Autodesk Inventor part; units mm, degrees
(part 2 of 3)
  line L952 (4.2416, 3.358) -> (4.3453, 3.3717)
  arc A20 (4.5494, 3.0907) -> (4.3453, 3.3717) centre (0, 0) ccw
  line L953 (4.5494, 3.0907) -> (4.5044, 2.9964)
  line L954 (4.5044, 2.9964) -> (4.4538, 2.9006)
  line L955 (4.4538, 2.9006) -> (4.403, 2.8135)
  line L956 (4.403, 2.8135) -> (4.3541, 2.7371)
  line L957 (4.3541, 2.7371) -> (4.3057, 2.6681)
  line L958 (4.3057, 2.6681) -> (4.2604, 2.609)
  line L959 (4.2604, 2.609) -> (4.2171, 2.5571)
  line L960 (4.2171, 2.5571) -> (4.1777, 2.5137)
  line L961 (4.1777, 2.5137) -> (4.1429, 2.4785)
  line L962 (4.1429, 2.4785) -> (4.0862, 2.4275)
  line L963 (4.0862, 2.4275) -> (4.0491, 2.3994)
  line L964 (4.0491, 2.3994) -> (3.9753, 2.3516)
  line L965 (3.9753, 2.3516) -> (3.9286, 2.314)
  line L966 (3.9286, 2.314) -> (3.9091, 2.2954)
  line L967 (3.9091, 2.2954) -> (3.892, 2.277)
  line L968 (3.892, 2.277) -> (3.8773, 2.2589)
  line L969 (3.8773, 2.2589) -> (3.8652, 2.2413)
  line L970 (3.8652, 2.2413) -> (3.8554, 2.2242)
  line L971 (3.8554, 2.2242) -> (3.8481, 2.2077)
  line L972 (3.8481, 2.2077) -> (3.8431, 2.1919)
  line L973 (3.8431, 2.1919) -> (3.8404, 2.1769)
  line L974 (3.8404, 2.1769) -> (3.8401, 2.1628)
  line L975 (3.8401, 2.1628) -> (3.842, 2.1497)
  line L976 (3.842, 2.1497) -> (3.8489, 2.1321)
  line L977 (3.8489, 2.1321) -> (3.9204, 1.9976)
  line L978 (3.9204, 1.9976) -> (3.9872, 1.8607)
  line L979 (3.9872, 1.8607) -> (3.9974, 1.8447)
  line L980 (3.9974, 1.8447) -> (4.0069, 1.8354)
  line L981 (4.0069, 1.8354) -> (4.0185, 1.8274)
  line L982 (4.0185, 1.8274) -> (4.0322, 1.8208)
  line L983 (4.0322, 1.8208) -> (4.0479, 1.8155)
  line L984 (4.0479, 1.8155) -> (4.0655, 1.8118)
  line L985 (4.0655, 1.8118) -> (4.0851, 1.8096)
  line L986 (4.0851, 1.8096) -> (4.1065, 1.8091)
  line L987 (4.1065, 1.8091) -> (4.1297, 1.8103)
  line L988 (4.1297, 1.8103) -> (4.1547, 1.8133)
  line L989 (4.1547, 1.8133) -> (4.1813, 1.8182)
  line L990 (4.1813, 1.8182) -> (4.2391, 1.8339)
  line L991 (4.2391, 1.8339) -> (4.3212, 1.8655)
  line L992 (4.3212, 1.8655) -> (4.3657, 1.879)
  line L993 (4.3657, 1.879) -> (4.4403, 1.8949)
  line L994 (4.4403, 1.8949) -> (4.4892, 1.9023)
  line L995 (4.4892, 1.9023) -> (4.5475, 1.9087)
  line L996 (4.5475, 1.9087) -> (4.6149, 1.9132)
  line L997 (4.6149, 1.9132) -> (4.6893, 1.9151)
  line L998 (4.6893, 1.9151) -> (4.7736, 1.9137)
  line L999 (4.7736, 1.9137) -> (4.8642, 1.9084)
  line L1000 (4.8642, 1.9084) -> (4.9645, 1.8983)
  line L1001 (4.9645, 1.8983) -> (5.0717, 1.8829)
  line L1002 (5.0717, 1.8829) -> (5.1745, 1.8639)
  arc A21 (5.2818, 1.5336) -> (5.1745, 1.8639) centre (0, 0) ccw
  line L1003 (5.2818, 1.5336) -> (5.2098, 1.4578)
  line L1004 (5.2098, 1.4578) -> (5.1322, 1.3823)
  line L1005 (5.1322, 1.3823) -> (5.0569, 1.3152)
  line L1006 (5.0569, 1.3152) -> (4.9868, 1.2577)
  line L1007 (4.9868, 1.2577) -> (4.9194, 1.207)
  line L1008 (4.9194, 1.207) -> (4.8581, 1.1647)
  line L1009 (4.8581, 1.1647) -> (4.8009, 1.1288)
  line L1010 (4.8009, 1.1288) -> (4.75, 1.0997)
  line L1011 (4.75, 1.0997) -> (4.7061, 1.0769)
  line L1012 (4.7061, 1.0769) -> (4.6364, 1.046)
  line L1013 (4.6364, 1.046) -> (4.5924, 1.0307)
  line L1014 (4.5924, 1.0307) -> (4.5075, 1.0081)
  line L1015 (4.5075, 1.0081) -> (4.4514, 0.9867)
  line L1016 (4.4514, 0.9867) -> (4.427, 0.9751)
  line L1017 (4.427, 0.9751) -> (4.4051, 0.9628)
  line L1018 (4.4051, 0.9628) -> (4.3856, 0.9502)
  line L1019 (4.3856, 0.9502) -> (4.3686, 0.9372)
  line L1020 (4.3686, 0.9372) -> (4.354, 0.9239)
  line L1021 (4.354, 0.9239) -> (4.3419, 0.9105)
  line L1022 (4.3419, 0.9105) -> (4.3323, 0.897)
  line L1023 (4.3323, 0.897) -> (4.3252, 0.8836)
  line L1024 (4.3252, 0.8836) -> (4.3205, 0.8703)
  line L1025 (4.3205, 0.8703) -> (4.3182, 0.8572)
  line L1026 (4.3182, 0.8572) -> (4.3194, 0.8383)
  line L1027 (4.3194, 0.8383) -> (4.3458, 0.6883)
  line L1028 (4.3458, 0.6883) -> (4.3671, 0.5375)
  line L1029 (4.3671, 0.5375) -> (4.3718, 0.5191)
  line L1030 (4.3718, 0.5191) -> (4.378, 0.5074)
  line L1031 (4.378, 0.5074) -> (4.3865, 0.4962)
  line L1032 (4.3865, 0.4962) -> (4.3975, 0.4856)
  line L1033 (4.3975, 0.4856) -> (4.4108, 0.4758)
  line L1034 (4.4108, 0.4758) -> (4.4264, 0.4668)
  line L1035 (4.4264, 0.4668) -> (4.4444, 0.4587)
  line L1036 (4.4444, 0.4587) -> (4.4646, 0.4516)
  line L1037 (4.4646, 0.4516) -> (4.487, 0.4455)
  line L1038 (4.487, 0.4455) -> (4.5117, 0.4407)
  line L1039 (4.5117, 0.4407) -> (4.5385, 0.4371)
  line L1040 (4.5385, 0.4371) -> (4.5984, 0.4341)
  line L1041 (4.5984, 0.4341) -> (4.6862, 0.4388)
  line L1042 (4.6862, 0.4388) -> (4.7327, 0.438)
  line L1043 (4.7327, 0.438) -> (4.8085, 0.43)
  line L1044 (4.8085, 0.43) -> (4.8574, 0.422)
  line L1045 (4.8574, 0.422) -> (4.9147, 0.41)
  line L1046 (4.9147, 0.41) -> (4.9802, 0.3935)
  line L1047 (4.9802, 0.3935) -> (5.0516, 0.3723)
  line L1048 (5.0516, 0.3723) -> (5.1313, 0.3449)
  line L1049 (5.1313, 0.3449) -> (5.2159, 0.3118)
  line L1050 (5.2159, 0.3118) -> (5.3081, 0.2712)
  line L1051 (5.3081, 0.2712) -> (5.4053, 0.2235)
  line L1052 (5.4053, 0.2235) -> (5.4973, 0.1736)
  arc A22 (5.4973, -0.1736) -> (5.4973, 0.1736) centre (0, 0) ccw
  line L1053 (5.4973, -0.1736) -> (5.4053, -0.2235)
  line L1054 (5.4053, -0.2235) -> (5.3081, -0.2712)
  line L1055 (5.3081, -0.2712) -> (5.2159, -0.3118)
  line L1056 (5.2159, -0.3118) -> (5.1313, -0.3449)
  line L1057 (5.1313, -0.3449) -> (5.0516, -0.3723)
  line L1058 (5.0516, -0.3723) -> (4.9802, -0.3935)
  line L1059 (4.9802, -0.3935) -> (4.9147, -0.41)
  line L1060 (4.9147, -0.41) -> (4.8574, -0.422)
  line L1061 (4.8574, -0.422) -> (4.8085, -0.43)
  line L1062 (4.8085, -0.43) -> (4.7327, -0.438)
  line L1063 (4.7327, -0.438) -> (4.6862, -0.4388)
  line L1064 (4.6862, -0.4388) -> (4.5984, -0.4341)
  line L1065 (4.5984, -0.4341) -> (4.5385, -0.4371)
  line L1066 (4.5385, -0.4371) -> (4.5117, -0.4407)
  line L1067 (4.5117, -0.4407) -> (4.487, -0.4455)
  line L1068 (4.487, -0.4455) -> (4.4646, -0.4516)
  line L1069 (4.4646, -0.4516) -> (4.4444, -0.4587)
  line L1070 (4.4444, -0.4587) -> (4.4264, -0.4668)
  line L1071 (4.4264, -0.4668) -> (4.4108, -0.4758)
  line L1072 (4.4108, -0.4758) -> (4.3975, -0.4856)
  line L1073 (4.3975, -0.4856) -> (4.3865, -0.4962)
  line L1074 (4.3865, -0.4962) -> (4.378, -0.5074)
  line L1075 (4.378, -0.5074) -> (4.3718, -0.5191)
  line L1076 (4.3718, -0.5191) -> (4.3671, -0.5375)
  line L1077 (4.3671, -0.5375) -> (4.3458, -0.6883)
  line L1078 (4.3458, -0.6883) -> (4.3194, -0.8383)
  line L1079 (4.3194, -0.8383) -> (4.3182, -0.8572)
  line L1080 (4.3182, -0.8572) -> (4.3205, -0.8703)
  line L1081 (4.3205, -0.8703) -> (4.3252, -0.8836)
  line L1082 (4.3252, -0.8836) -> (4.3323, -0.897)
  line L1083 (4.3323, -0.897) -> (4.3419, -0.9105)
  line L1084 (4.3419, -0.9105) -> (4.354, -0.9239)
  line L1085 (4.354, -0.9239) -> (4.3686, -0.9372)
  line L1086 (4.3686, -0.9372) -> (4.3856, -0.9502)
  line L1087 (4.3856, -0.9502) -> (4.4051, -0.9628)
  line L1088 (4.4051, -0.9628) -> (4.427, -0.9751)
  line L1089 (4.427, -0.9751) -> (4.4514, -0.9867)
  line L1090 (4.4514, -0.9867) -> (4.5075, -1.0081)
  line L1091 (4.5075, -1.0081) -> (4.5924, -1.0307)
  line L1092 (4.5924, -1.0307) -> (4.6364, -1.046)
  line L1093 (4.6364, -1.046) -> (4.7061, -1.0769)
  line L1094 (4.7061, -1.0769) -> (4.75, -1.0997)
  line L1095 (4.75, -1.0997) -> (4.8009, -1.1288)
  line L1096 (4.8009, -1.1288) -> (4.8581, -1.1647)
  line L1097 (4.8581, -1.1647) -> (4.9194, -1.207)
  line L1098 (4.9194, -1.207) -> (4.9868, -1.2577)
  line L1099 (4.9868, -1.2577) -> (5.0569, -1.3152)
  line L1100 (5.0569, -1.3152) -> (5.1322, -1.3823)
  line L1101 (5.1322, -1.3823) -> (5.2098, -1.4578)
  line L1102 (5.2098, -1.4578) -> (5.2818, -1.5336)
  arc A23 (5.1745, -1.8639) -> (5.2818, -1.5336) centre (0, 0) ccw
  line L1103 (5.1745, -1.8639) -> (5.0717, -1.8829)
  line L1104 (5.0717, -1.8829) -> (4.9645, -1.8983)
  line L1105 (4.9645, -1.8983) -> (4.8642, -1.9084)
  line L1106 (4.8642, -1.9084) -> (4.7736, -1.9137)
  line L1107 (4.7736, -1.9137) -> (4.6893, -1.9151)
  line L1108 (4.6893, -1.9151) -> (4.6149, -1.9132)
  line L1109 (4.6149, -1.9132) -> (4.5475, -1.9087)
  line L1110 (4.5475, -1.9087) -> (4.4892, -1.9023)
  line L1111 (4.4892, -1.9023) -> (4.4403, -1.8949)
  line L1112 (4.4403, -1.8949) -> (4.3657, -1.879)
  line L1113 (4.3657, -1.879) -> (4.3212, -1.8655)
  line L1114 (4.3212, -1.8655) -> (4.2391, -1.8339)
  line L1115 (4.2391, -1.8339) -> (4.1813, -1.8182)
  line L1116 (4.1813, -1.8182) -> (4.1547, -1.8133)
  line L1117 (4.1547, -1.8133) -> (4.1297, -1.8103)
  line L1118 (4.1297, -1.8103) -> (4.1065, -1.8091)
  line L1119 (4.1065, -1.8091) -> (4.0851, -1.8096)
  line L1120 (4.0851, -1.8096) -> (4.0655, -1.8118)
  line L1121 (4.0655, -1.8118) -> (4.0479, -1.8155)
  line L1122 (4.0479, -1.8155) -> (4.0322, -1.8208)
  line L1123 (4.0322, -1.8208) -> (4.0185, -1.8274)
  line L1124 (4.0185, -1.8274) -> (4.0069, -1.8354)
  line L1125 (4.0069, -1.8354) -> (3.9974, -1.8447)
  line L1126 (3.9974, -1.8447) -> (3.9872, -1.8607)
  line L1127 (3.9872, -1.8607) -> (3.9204, -1.9976)
  line L1128 (3.9204, -1.9976) -> (3.8489, -2.1321)
  line L1129 (3.8489, -2.1321) -> (3.842, -2.1497)
  line L1130 (3.842, -2.1497) -> (3.8401, -2.1628)
  line L1131 (3.8401, -2.1628) -> (3.8404, -2.1769)
  line L1132 (3.8404, -2.1769) -> (3.8431, -2.1919)
  line L1133 (3.8431, -2.1919) -> (3.8481, -2.2077)
  line L1134 (3.8481, -2.2077) -> (3.8554, -2.2242)
  line L1135 (3.8554, -2.2242) -> (3.8652, -2.2413)
  line L1136 (3.8652, -2.2413) -> (3.8773, -2.2589)
  line L1137 (3.8773, -2.2589) -> (3.892, -2.277)
  line L1138 (3.892, -2.277) -> (3.9091, -2.2954)
  line L1139 (3.9091, -2.2954) -> (3.9286, -2.314)
  line L1140 (3.9286, -2.314) -> (3.9753, -2.3516)
  line L1141 (3.9753, -2.3516) -> (4.0491, -2.3994)
  line L1142 (4.0491, -2.3994) -> (4.0862, -2.4275)
  line L1143 (4.0862, -2.4275) -> (4.1429, -2.4785)
  line L1144 (4.1429, -2.4785) -> (4.1777, -2.5137)
  line L1145 (4.1777, -2.5137) -> (4.2171, -2.5571)
  line L1146 (4.2171, -2.5571) -> (4.2604, -2.609)
  line L1147 (4.2604, -2.609) -> (4.3057, -2.6681)
  line L1148 (4.3057, -2.6681) -> (4.3541, -2.7371)
  line L1149 (4.3541, -2.7371) -> (4.403, -2.8135)
  line L1150 (4.403, -2.8135) -> (4.4538, -2.9006)
  line L1151 (4.4538, -2.9006) -> (4.5044, -2.9964)
  line L1152 (4.5044, -2.9964) -> (4.5494, -3.0907)
  arc A24 (4.3453, -3.3717) -> (4.5494, -3.0907) centre (0, 0) ccw
  line L1153 (4.3453, -3.3717) -> (4.2416, -3.358)
  line L1154 (4.2416, -3.358) -> (4.1349, -3.3395)
  line L1155 (4.1349, -3.3395) -> (4.0364, -3.3181)
  line L1156 (4.0364, -3.3181) -> (3.9486, -3.2952)
  line L1157 (3.9486, -3.2952) -> (3.868, -3.2704)
  line L1158 (3.868, -3.2704) -> (3.7978, -3.2457)
  line L1159 (3.7978, -3.2457) -> (3.7351, -3.2205)
  line L1160 (3.7351, -3.2205) -> (3.6817, -3.1965)
  line L1161 (3.6817, -3.1965) -> (3.6374, -3.1743)
  line L1162 (3.6374, -3.1743) -> (3.5714, -3.1361)
  line L1163 (3.5714, -3.1361) -> (3.5332, -3.1095)
  line L1164 (3.5332, -3.1095) -> (3.465, -3.0541)
  line L1165 (3.465, -3.0541) -> (3.4148, -3.0213)
  line L1166 (3.4148, -3.0213) -> (3.391, -3.0084)
  line L1167 (3.391, -3.0084) -> (3.3682, -2.9979)
  line L1168 (3.3682, -2.9979) -> (3.3465, -2.9895)
  line L1169 (3.3465, -2.9895) -> (3.326, -2.9834)
  line L1170 (3.326, -2.9834) -> (3.3067, -2.9794)
  line L1171 (3.3067, -2.9794) -> (3.2887, -2.9775)
  line L1172 (3.2887, -2.9775) -> (3.2722, -2.9777)
  line L1173 (3.2722, -2.9777) -> (3.2571, -2.9798)
  line L1174 (3.2571, -2.9798) -> (3.2436, -2.9838)
  line L1175 (3.2436, -2.9838) -> (3.2317, -2.9896)
  line L1176 (3.2317, -2.9896) -> (3.2171, -3.0017)
  line L1177 (3.2171, -3.0017) -> (3.1113, -3.1113)
  line L1178 (3.1113, -3.1113) -> (3.0017, -3.2171)
  line L1179 (3.0017, -3.2171) -> (2.9896, -3.2317)
  line L1180 (2.9896, -3.2317) -> (2.9838, -3.2436)
  line L1181 (2.9838, -3.2436) -> (2.9798, -3.2571)
  line L1182 (2.9798, -3.2571) -> (2.9777, -3.2722)
  line L1183 (2.9777, -3.2722) -> (2.9775, -3.2887)
  line L1184 (2.9775, -3.2887) -> (2.9794, -3.3067)
  line L1185 (2.9794, -3.3067) -> (2.9834, -3.326)
  line L1186 (2.9834, -3.326) -> (2.9895, -3.3465)
  line L1187 (2.9895, -3.3465) -> (2.9979, -3.3682)
  line L1188 (2.9979, -3.3682) -> (3.0084, -3.391)
  line L1189 (3.0084, -3.391) -> (3.0213, -3.4148)
  line L1190 (3.0213, -3.4148) -> (3.0541, -3.465)
  line L1191 (3.0541, -3.465) -> (3.1095, -3.5332)
  line L1192 (3.1095, -3.5332) -> (3.1361, -3.5714)
  line L1193 (3.1361, -3.5714) -> (3.1743, -3.6374)
  line L1194 (3.1743, -3.6374) -> (3.1965, -3.6817)
  line L1195 (3.1965, -3.6817) -> (3.2205, -3.7351)
  line L1196 (3.2205, -3.7351) -> (3.2457, -3.7978)
  line L1197 (3.2457, -3.7978) -> (3.2704, -3.868)
  line L1198 (3.2704, -3.868) -> (3.2952, -3.9486)
  line L1199 (3.2952, -3.9486) -> (3.3181, -4.0364)
  line L1200 (3.3181, -4.0364) -> (3.3395, -4.1349)
  line L1201 (3.3395, -4.1349) -> (3.358, -4.2416)
  line L1202 (3.358, -4.2416) -> (3.3717, -4.3453)
  arc A25 (3.0907, -4.5494) -> (3.3717, -4.3453) centre (0, 0) ccw
  line L1203 (3.0907, -4.5494) -> (2.9964, -4.5044)
  line L1204 (2.9964, -4.5044) -> (2.9006, -4.4538)
  line L1205 (2.9006, -4.4538) -> (2.8135, -4.403)
  line L1206 (2.8135, -4.403) -> (2.7371, -4.3541)
  line L1207 (2.7371, -4.3541) -> (2.6681, -4.3057)
  line L1208 (2.6681, -4.3057) -> (2.609, -4.2604)
  line L1209 (2.609, -4.2604) -> (2.5571, -4.2171)
  line L1210 (2.5571, -4.2171) -> (2.5137, -4.1777)
  line L1211 (2.5137, -4.1777) -> (2.4785, -4.1429)
  line L1212 (2.4785, -4.1429) -> (2.4275, -4.0862)
  line L1213 (2.4275, -4.0862) -> (2.3994, -4.0491)
  line L1214 (2.3994, -4.0491) -> (2.3516, -3.9753)
  line L1215 (2.3516, -3.9753) -> (2.314, -3.9286)
  line L1216 (2.314, -3.9286) -> (2.2954, -3.9091)
  line L1217 (2.2954, -3.9091) -> (2.277, -3.892)
  line L1218 (2.277, -3.892) -> (2.2589, -3.8773)
  line L1219 (2.2589, -3.8773) -> (2.2413, -3.8652)
  line L1220 (2.2413, -3.8652) -> (2.2242, -3.8554)
  line L1221 (2.2242, -3.8554) -> (2.2077, -3.8481)
  line L1222 (2.2077, -3.8481) -> (2.1919, -3.8431)
  line L1223 (2.1919, -3.8431) -> (2.1769, -3.8404)
  line L1224 (2.1769, -3.8404) -> (2.1628, -3.8401)
  line L1225 (2.1628, -3.8401) -> (2.1497, -3.842)
  line L1226 (2.1497, -3.842) -> (2.1321, -3.8489)
  line L1227 (2.1321, -3.8489) -> (1.9976, -3.9204)
  line L1228 (1.9976, -3.9204) -> (1.8607, -3.9872)
  line L1229 (1.8607, -3.9872) -> (1.8447, -3.9974)
  line L1230 (1.8447, -3.9974) -> (1.8354, -4.0069)
  line L1231 (1.8354, -4.0069) -> (1.8274, -4.0185)
  line L1232 (1.8274, -4.0185) -> (1.8208, -4.0322)
  line L1233 (1.8208, -4.0322) -> (1.8155, -4.0479)
  line L1234 (1.8155, -4.0479) -> (1.8118, -4.0655)
  line L1235 (1.8118, -4.0655) -> (1.8096, -4.0851)
  line L1236 (1.8096, -4.0851) -> (1.8091, -4.1065)
  line L1237 (1.8091, -4.1065) -> (1.8103, -4.1297)
  line L1238 (1.8103, -4.1297) -> (1.8133, -4.1547)
  line L1239 (1.8133, -4.1547) -> (1.8182, -4.1813)
  line L1240 (1.8182, -4.1813) -> (1.8339, -4.2391)
  line L1241 (1.8339, -4.2391) -> (1.8655, -4.3212)
  line L1242 (1.8655, -4.3212) -> (1.879, -4.3657)
  line L1243 (1.879, -4.3657) -> (1.8949, -4.4403)
  line L1244 (1.8949, -4.4403) -> (1.9023, -4.4892)
  line L1245 (1.9023, -4.4892) -> (1.9087, -4.5475)
  line L1246 (1.9087, -4.5475) -> (1.9132, -4.6149)
  line L1247 (1.9132, -4.6149) -> (1.9151, -4.6893)
  line L1248 (1.9151, -4.6893) -> (1.9137, -4.7736)
  line L1249 (1.9137, -4.7736) -> (1.9084, -4.8642)
  line L1250 (1.9084, -4.8642) -> (1.8983, -4.9645)
  line L1251 (1.8983, -4.9645) -> (1.8829, -5.0717)
  line L1252 (1.8829, -5.0717) -> (1.8639, -5.1745)
  arc A26 (1.5336, -5.2818) -> (1.8639, -5.1745) centre (0, 0) ccw
  line L1253 (1.5336, -5.2818) -> (1.4578, -5.2098)
  line L1254 (1.4578, -5.2098) -> (1.3823, -5.1322)
  line L1255 (1.3823, -5.1322) -> (1.3152, -5.0569)
  line L1256 (1.3152, -5.0569) -> (1.2577, -4.9868)
  line L1257 (1.2577, -4.9868) -> (1.207, -4.9194)
  line L1258 (1.207, -4.9194) -> (1.1647, -4.8581)
  line L1259 (1.1647, -4.8581) -> (1.1288, -4.8009)
  line L1260 (1.1288, -4.8009) -> (1.0997, -4.75)
  line L1261 (1.0997, -4.75) -> (1.0769, -4.7061)
  line L1262 (1.0769, -4.7061) -> (1.046, -4.6364)
  line L1263 (1.046, -4.6364) -> (1.0307, -4.5924)
  line L1264 (1.0307, -4.5924) -> (1.0081, -4.5075)
  line L1265 (1.0081, -4.5075) -> (0.9867, -4.4514)
  line L1266 (0.9867, -4.4514) -> (0.9751, -4.427)
  line L1267 (0.9751, -4.427) -> (0.9628, -4.4051)
  line L1268 (0.9628, -4.4051) -> (0.9502, -4.3856)
  line L1269 (0.9502, -4.3856) -> (0.9372, -4.3686)
  line L1270 (0.9372, -4.3686) -> (0.9239, -4.354)
  line L1271 (0.9239, -4.354) -> (0.9105, -4.3419)
  line L1272 (0.9105, -4.3419) -> (0.897, -4.3323)
  line L1273 (0.897, -4.3323) -> (0.8836, -4.3252)
  line L1274 (0.8836, -4.3252) -> (0.8703, -4.3205)
  line L1275 (0.8703, -4.3205) -> (0.8572, -4.3182)
  line L1276 (0.8572, -4.3182) -> (0.8383, -4.3194)
  line L1277 (0.8383, -4.3194) -> (0.6883, -4.3458)
  line L1278 (0.6883, -4.3458) -> (0.5375, -4.3671)
  line L1279 (0.5375, -4.3671) -> (0.5191, -4.3718)
  line L1280 (0.5191, -4.3718) -> (0.5074, -4.378)
  line L1281 (0.5074, -4.378) -> (0.4962, -4.3865)
  line L1282 (0.4962, -4.3865) -> (0.4856, -4.3975)
  line L1283 (0.4856, -4.3975) -> (0.4758, -4.4108)
  line L1284 (0.4758, -4.4108) -> (0.4668, -4.4264)
  line L1285 (0.4668, -4.4264) -> (0.4587, -4.4444)
  line L1286 (0.4587, -4.4444) -> (0.4516, -4.4646)
  line L1287 (0.4516, -4.4646) -> (0.4455, -4.487)
  line L1288 (0.4455, -4.487) -> (0.4407, -4.5117)
  line L1289 (0.4407, -4.5117) -> (0.4371, -4.5385)
  line L1290 (0.4371, -4.5385) -> (0.4341, -4.5984)
  line L1291 (0.4341, -4.5984) -> (0.4388, -4.6862)
  line L1292 (0.4388, -4.6862) -> (0.438, -4.7327)
  line L1293 (0.438, -4.7327) -> (0.43, -4.8085)
  line L1294 (0.43, -4.8085) -> (0.422, -4.8574)
  line L1295 (0.422, -4.8574) -> (0.41, -4.9147)
  line L1296 (0.41, -4.9147) -> (0.3935, -4.9802)
  line L1297 (0.3935, -4.9802) -> (0.3723, -5.0516)
  line L1298 (0.3723, -5.0516) -> (0.3449, -5.1313)
  line L1299 (0.3449, -5.1313) -> (0.3118, -5.2159)
  line L1300 (0.3118, -5.2159) -> (0.2712, -5.3081)
  line L1301 (0.2712, -5.3081) -> (0.2235, -5.4053)
  line L1302 (0.2235, -5.4053) -> (0.1736, -5.4973)
  arc A27 (-0.1736, -5.4973) -> (0.1736, -5.4973) centre (0, 0) ccw
  line L1303 (-0.1736, -5.4973) -> (-0.2235, -5.4053)
  line L1304 (-0.2235, -5.4053) -> (-0.2712, -5.3081)
  line L1305 (-0.2712, -5.3081) -> (-0.3118, -5.2159)
  line L1306 (-0.3118, -5.2159) -> (-0.3449, -5.1313)
  line L1307 (-0.3449, -5.1313) -> (-0.3723, -5.0516)
  line L1308 (-0.3723, -5.0516) -> (-0.3935, -4.9802)
  line L1309 (-0.3935, -4.9802) -> (-0.41, -4.9147)
  line L1310 (-0.41, -4.9147) -> (-0.422, -4.8574)
  line L1311 (-0.422, -4.8574) -> (-0.43, -4.8085)
  line L1312 (-0.43, -4.8085) -> (-0.438, -4.7327)
  line L1313 (-0.438, -4.7327) -> (-0.4388, -4.6862)
  line L1314 (-0.4388, -4.6862) -> (-0.4341, -4.5984)
  line L1315 (-0.4341, -4.5984) -> (-0.4371, -4.5385)
  line L1316 (-0.4371, -4.5385) -> (-0.4407, -4.5117)
  line L1317 (-0.4407, -4.5117) -> (-0.4455, -4.487)
  line L1318 (-0.4455, -4.487) -> (-0.4516, -4.4646)
  line L1319 (-0.4516, -4.4646) -> (-0.4587, -4.4444)
  line L1320 (-0.4587, -4.4444) -> (-0.4668, -4.4264)
  line L1321 (-0.4668, -4.4264) -> (-0.4758, -4.4108)
  line L1322 (-0.4758, -4.4108) -> (-0.4856, -4.3975)
  line L1323 (-0.4856, -4.3975) -> (-0.4962, -4.3865)
  line L1324 (-0.4962, -4.3865) -> (-0.5074, -4.378)
  line L1325 (-0.5074, -4.378) -> (-0.5191, -4.3718)
  line L1326 (-0.5191, -4.3718) -> (-0.5375, -4.3671)
  line L1327 (-0.5375, -4.3671) -> (-0.6883, -4.3458)
  line L1328 (-0.6883, -4.3458) -> (-0.8383, -4.3194)
  line L1329 (-0.8383, -4.3194) -> (-0.8572, -4.3182)
  line L1330 (-0.8572, -4.3182) -> (-0.8703, -4.3205)
  line L1331 (-0.8703, -4.3205) -> (-0.8836, -4.3252)
  line L1332 (-0.8836, -4.3252) -> (-0.897, -4.3323)
  line L1333 (-0.897, -4.3323) -> (-0.9105, -4.3419)
  line L1334 (-0.9105, -4.3419) -> (-0.9239, -4.354)
  line L1335 (-0.9239, -4.354) -> (-0.9372, -4.3686)
  line L1336 (-0.9372, -4.3686) -> (-0.9502, -4.3856)
  line L1337 (-0.9502, -4.3856) -> (-0.9628, -4.4051)
  line L1338 (-0.9628, -4.4051) -> (-0.9751, -4.427)
  line L1339 (-0.9751, -4.427) -> (-0.9867, -4.4514)
  line L1340 (-0.9867, -4.4514) -> (-1.0081, -4.5075)
  line L1341 (-1.0081, -4.5075) -> (-1.0307, -4.5924)
  line L1342 (-1.0307, -4.5924) -> (-1.046, -4.6364)
  line L1343 (-1.046, -4.6364) -> (-1.0769, -4.7061)
  line L1344 (-1.0769, -4.7061) -> (-1.0997, -4.75)
  line L1345 (-1.0997, -4.75) -> (-1.1288, -4.8009)
  line L1346 (-1.1288, -4.8009) -> (-1.1647, -4.8581)
  line L1347 (-1.1647, -4.8581) -> (-1.207, -4.9194)
  line L1348 (-1.207, -4.9194) -> (-1.2577, -4.9868)
  line L1349 (-1.2577, -4.9868) -> (-1.3152, -5.0569)
  line L1350 (-1.3152, -5.0569) -> (-1.3823, -5.1322)
  line L1351 (-1.3823, -5.1322) -> (-1.4578, -5.2098)
  line L1352 (-1.4578, -5.2098) -> (-1.5336, -5.2818)
  arc A28 (-1.8639, -5.1745) -> (-1.5336, -5.2818) centre (0, 0) ccw
  line L1353 (-1.8639, -5.1745) -> (-1.8829, -5.0717)
  line L1354 (-1.8829, -5.0717) -> (-1.8983, -4.9645)
  line L1355 (-1.8983, -4.9645) -> (-1.9084, -4.8642)
  line L1356 (-1.9084, -4.8642) -> (-1.9137, -4.7736)
  line L1357 (-1.9137, -4.7736) -> (-1.9151, -4.6893)
  line L1358 (-1.9151, -4.6893) -> (-1.9132, -4.6149)
  line L1359 (-1.9132, -4.6149) -> (-1.9087, -4.5475)
  line L1360 (-1.9087, -4.5475) -> (-1.9023, -4.4892)
  line L1361 (-1.9023, -4.4892) -> (-1.8949, -4.4403)
  line L1362 (-1.8949, -4.4403) -> (-1.879, -4.3657)
  line L1363 (-1.879, -4.3657) -> (-1.8655, -4.3212)
  line L1364 (-1.8655, -4.3212) -> (-1.8339, -4.2391)
  line L1365 (-1.8339, -4.2391) -> (-1.8182, -4.1813)
  line L1366 (-1.8182, -4.1813) -> (-1.8133, -4.1547)
  line L1367 (-1.8133, -4.1547) -> (-1.8103, -4.1297)
  line L1368 (-1.8103, -4.1297) -> (-1.8091, -4.1065)
  line L1369 (-1.8091, -4.1065) -> (-1.8096, -4.0851)
  line L1370 (-1.8096, -4.0851) -> (-1.8118, -4.0655)
  line L1371 (-1.8118, -4.0655) -> (-1.8155, -4.0479)
  line L1372 (-1.8155, -4.0479) -> (-1.8208, -4.0322)
  line L1373 (-1.8208, -4.0322) -> (-1.8274, -4.0185)
  line L1374 (-1.8274, -4.0185) -> (-1.8354, -4.0069)
  line L1375 (-1.8354, -4.0069) -> (-1.8447, -3.9974)
  line L1376 (-1.8447, -3.9974) -> (-1.8607, -3.9872)
  line L1377 (-1.8607, -3.9872) -> (-1.9976, -3.9204)
  line L1378 (-1.9976, -3.9204) -> (-2.1321, -3.8489)
  line L1379 (-2.1321, -3.8489) -> (-2.1497, -3.842)
  line L1380 (-2.1497, -3.842) -> (-2.1628, -3.8401)
  line L1381 (-2.1628, -3.8401) -> (-2.1769, -3.8404)
  line L1382 (-2.1769, -3.8404) -> (-2.1919, -3.8431)
  line L1383 (-2.1919, -3.8431) -> (-2.2077, -3.8481)
  line L1384 (-2.2077, -3.8481) -> (-2.2242, -3.8554)
  line L1385 (-2.2242, -3.8554) -> (-2.2413, -3.8652)
  line L1386 (-2.2413, -3.8652) -> (-2.2589, -3.8773)
  line L1387 (-2.2589, -3.8773) -> (-2.277, -3.892)
  line L1388 (-2.277, -3.892) -> (-2.2954, -3.9091)
  line L1389 (-2.2954, -3.9091) -> (-2.314, -3.9286)
  line L1390 (-2.314, -3.9286) -> (-2.3516, -3.9753)
  line L1391 (-2.3516, -3.9753) -> (-2.3994, -4.0491)
  line L1392 (-2.3994, -4.0491) -> (-2.4275, -4.0862)
  line L1393 (-2.4275, -4.0862) -> (-2.4785, -4.1429)
  line L1394 (-2.4785, -4.1429) -> (-2.5137, -4.1777)
  line L1395 (-2.5137, -4.1777) -> (-2.5571, -4.2171)
  line L1396 (-2.5571, -4.2171) -> (-2.609, -4.2604)
  line L1397 (-2.609, -4.2604) -> (-2.6681, -4.3057)
  line L1398 (-2.6681, -4.3057) -> (-2.7371, -4.3541)
  line L1399 (-2.7371, -4.3541) -> (-2.8135, -4.403)
  line L1400 (-2.8135, -4.403) -> (-2.9006, -4.4538)
  line L1401 (-2.9006, -4.4538) -> (-2.9964, -4.5044)
  line L1402 (-2.9964, -4.5044) -> (-3.0907, -4.5494)
  arc A29 (-3.3717, -4.3453) -> (-3.0907, -4.5494) centre (0, 0) ccw
  line L1403 (-3.3717, -4.3453) -> (-3.358, -4.2416)
  line L1404 (-3.358, -4.2416) -> (-3.3395, -4.1349)
  line L1405 (-3.3395, -4.1349) -> (-3.3181, -4.0364)
  line L1406 (-3.3181, -4.0364) -> (-3.2952, -3.9486)
  line L1407 (-3.2952, -3.9486) -> (-3.2704, -3.868)
  line L1408 (-3.2704, -3.868) -> (-3.2457, -3.7978)
  line L1409 (-3.2457, -3.7978) -> (-3.2205, -3.7351)
  line L1410 (-3.2205, -3.7351) -> (-3.1965, -3.6817)
  line L1411 (-3.1965, -3.6817) -> (-3.1743, -3.6374)
  line L1412 (-3.1743, -3.6374) -> (-3.1361, -3.5714)
  line L1413 (-3.1361, -3.5714) -> (-3.1095, -3.5332)
  line L1414 (-3.1095, -3.5332) -> (-3.0541, -3.465)
  line L1415 (-3.0541, -3.465) -> (-3.0213, -3.4148)
  line L1416 (-3.0213, -3.4148) -> (-3.0084, -3.391)
  line L1417 (-3.0084, -3.391) -> (-2.9979, -3.3682)
  line L1418 (-2.9979, -3.3682) -> (-2.9895, -3.3465)
  line L1419 (-2.9895, -3.3465) -> (-2.9834, -3.326)
  line L1420 (-2.9834, -3.326) -> (-2.9794, -3.3067)
  line L1421 (-2.9794, -3.3067) -> (-2.9775, -3.2887)
  line L1422 (-2.9775, -3.2887) -> (-2.9777, -3.2722)
  line L1423 (-2.9777, -3.2722) -> (-2.9798, -3.2571)
  line L1424 (-2.9798, -3.2571) -> (-2.9838, -3.2436)
  line L1425 (-2.9838, -3.2436) -> (-2.9896, -3.2317)
  line L1426 (-2.9896, -3.2317) -> (-3.0017, -3.2171)
  line L1427 (-3.0017, -3.2171) -> (-3.1113, -3.1113)
  line L1428 (-3.1113, -3.1113) -> (-3.2171, -3.0017)
  line L1429 (-3.2171, -3.0017) -> (-3.2317, -2.9896)
  line L1430 (-3.2317, -2.9896) -> (-3.2436, -2.9838)
  line L1431 (-3.2436, -2.9838) -> (-3.2571, -2.9798)
  line L1432 (-3.2571, -2.9798) -> (-3.2722, -2.9777)
  line L1433 (-3.2722, -2.9777) -> (-3.2887, -2.9775)
  line L1434 (-3.2887, -2.9775) -> (-3.3067, -2.9794)
  line L1435 (-3.3067, -2.9794) -> (-3.326, -2.9834)
  line L1436 (-3.326, -2.9834) -> (-3.3465, -2.9895)
  line L1437 (-3.3465, -2.9895) -> (-3.3682, -2.9979)
  line L1438 (-3.3682, -2.9979) -> (-3.391, -3.0084)
  line L1439 (-3.391, -3.0084) -> (-3.4148, -3.0213)
  line L1440 (-3.4148, -3.0213) -> (-3.465, -3.0541)
  line L1441 (-3.465, -3.0541) -> (-3.5332, -3.1095)
  line L1442 (-3.5332, -3.1095) -> (-3.5714, -3.1361)
  line L1443 (-3.5714, -3.1361) -> (-3.6374, -3.1743)
  line L1444 (-3.6374, -3.1743) -> (-3.6817, -3.1965)
  line L1445 (-3.6817, -3.1965) -> (-3.7351, -3.2205)
  line L1446 (-3.7351, -3.2205) -> (-3.7978, -3.2457)
  line L1447 (-3.7978, -3.2457) -> (-3.868, -3.2704)
  line L1448 (-3.868, -3.2704) -> (-3.9486, -3.2952)
  line L1449 (-3.9486, -3.2952) -> (-4.0364, -3.3181)
  line L1450 (-4.0364, -3.3181) -> (-4.1349, -3.3395)
  line L1451 (-4.1349, -3.3395) -> (-4.2416, -3.358)
  line L1452 (-4.2416, -3.358) -> (-4.3453, -3.3717)
  arc A30 (-4.5494, -3.0907) -> (-4.3453, -3.3717) centre (0, 0) ccw
  line L1453 (-4.5494, -3.0907) -> (-4.5044, -2.9964)
  line L1454 (-4.5044, -2.9964) -> (-4.4538, -2.9006)
  line L1455 (-4.4538, -2.9006) -> (-4.403, -2.8135)
  line L1456 (-4.403, -2.8135) -> (-4.3541, -2.7371)
  line L1457 (-4.3541, -2.7371) -> (-4.3057, -2.6681)
  line L1458 (-4.3057, -2.6681) -> (-4.2604, -2.609)
  line L1459 (-4.2604, -2.609) -> (-4.2171, -2.5571)
  line L1460 (-4.2171, -2.5571) -> (-4.1777, -2.5137)
  line L1461 (-4.1777, -2.5137) -> (-4.1429, -2.4785)
  line L1462 (-4.1429, -2.4785) -> (-4.0862, -2.4275)
  line L1463 (-4.0862, -2.4275) -> (-4.0491, -2.3994)
  line L1464 (-4.0491, -2.3994) -> (-3.9753, -2.3516)
  line L1465 (-3.9753, -2.3516) -> (-3.9286, -2.314)
  line L1466 (-3.9286, -2.314) -> (-3.9091, -2.2954)
  line L1467 (-3.9091, -2.2954) -> (-3.892, -2.277)
  line L1468 (-3.892, -2.277) -> (-3.8773, -2.2589)
  line L1469 (-3.8773, -2.2589) -> (-3.8652, -2.2413)
  line L1470 (-3.8652, -2.2413) -> (-3.8554, -2.2242)
  line L1471 (-3.8554, -2.2242) -> (-3.8481, -2.2077)
  line L1472 (-3.8481, -2.2077) -> (-3.8431, -2.1919)
  line L1473 (-3.8431, -2.1919) -> (-3.8404, -2.1769)
  line L1474 (-3.8404, -2.1769) -> (-3.8401, -2.1628)
  line L1475 (-3.8401, -2.1628) -> (-3.842, -2.1497)
  line L1476 (-3.842, -2.1497) -> (-3.8489, -2.1321)
  line L1477 (-3.8489, -2.1321) -> (-3.9204, -1.9976)
  line L1478 (-3.9204, -1.9976) -> (-3.9872, -1.8607)
  line L1479 (-3.9872, -1.8607) -> (-3.9974, -1.8447)
  line L1480 (-3.9974, -1.8447) -> (-4.0069, -1.8354)
  line L1481 (-4.0069, -1.8354) -> (-4.0185, -1.8274)
  line L1482 (-4.0185, -1.8274) -> (-4.0322, -1.8208)
  line L1483 (-4.0322, -1.8208) -> (-4.0479, -1.8155)
  line L1484 (-4.0479, -1.8155) -> (-4.0655, -1.8118)
  line L1485 (-4.0655, -1.8118) -> (-4.0851, -1.8096)
  line L1486 (-4.0851, -1.8096) -> (-4.1065, -1.8091)
  line L1487 (-4.1065, -1.8091) -> (-4.1297, -1.8103)
  line L1488 (-4.1297, -1.8103) -> (-4.1547, -1.8133)
  line L1489 (-4.1547, -1.8133) -> (-4.1813, -1.8182)
  line L1490 (-4.1813, -1.8182) -> (-4.2391, -1.8339)
  line L1491 (-4.2391, -1.8339) -> (-4.3212, -1.8655)
  line L1492 (-4.3212, -1.8655) -> (-4.3657, -1.879)
  line L1493 (-4.3657, -1.879) -> (-4.4403, -1.8949)
  line L1494 (-4.4403, -1.8949) -> (-4.4892, -1.9023)
  line L1495 (-4.4892, -1.9023) -> (-4.5475, -1.9087)
  line L1496 (-4.5475, -1.9087) -> (-4.6149, -1.9132)
  line L1497 (-4.6149, -1.9132) -> (-4.6893, -1.9151)
  line L1498 (-4.6893, -1.9151) -> (-4.7736, -1.9137)
  line L1499 (-4.7736, -1.9137) -> (-4.8642, -1.9084)
  line L1500 (-4.8642, -1.9084) -> (-4.9645, -1.8983)
  line L1501 (-4.9645, -1.8983) -> (-5.0717, -1.8829)
  line L1502 (-5.0717, -1.8829) -> (-5.1745, -1.8639)
  arc A31 (-5.2818, -1.5336) -> (-5.1745, -1.8639) centre (0, 0) ccw
  line L1503 (5.2098, 1.4578) -> (5.1322, 1.3823)
  line L1504 (-5.2098, -1.4578) -> (-5.1322, -1.3823)
  line L1505 (-5.1322, -1.3823) -> (-5.0569, -1.3152)
  line L1506 (-5.0569, -1.3152) -> (-4.9868, -1.2577)
  line L1507 (-4.9868, -1.2577) -> (-4.9194, -1.207)
  line L1508 (-4.9194, -1.207) -> (-4.8581, -1.1647)
  line L1509 (-4.8581, -1.1647) -> (-4.8009, -1.1288)
  line L1510 (-4.8009, -1.1288) -> (-4.75, -1.0997)
  line L1511 (-4.75, -1.0997) -> (-4.7061, -1.0769)
  line L1512 (-4.7061, -1.0769) -> (-4.6364, -1.046)
  line L1513 (-4.6364, -1.046) -> (-4.5924, -1.0307)
  line L1514 (-4.5924, -1.0307) -> (-4.5075, -1.0081)
  line L1515 (-4.5075, -1.0081) -> (-4.4514, -0.9867)
  line L1516 (-4.4514, -0.9867) -> (-4.427, -0.9751)
  line L1517 (-4.427, -0.9751) -> (-4.4051, -0.9628)
  line L1518 (-4.4051, -0.9628) -> (-4.3856, -0.9502)
  line L1519 (-4.3856, -0.9502) -> (-4.3686, -0.9372)
  line L1520 (-4.3686, -0.9372) -> (-4.354, -0.9239)
  line L1521 (-4.354, -0.9239) -> (-4.3419, -0.9105)
  line L1522 (-4.3419, -0.9105) -> (-4.3323, -0.897)
  line L1523 (-4.3323, -0.897) -> (-4.3252, -0.8836)
  line L1524 (-4.3252, -0.8836) -> (-4.3205, -0.8703)
  line L1525 (-4.3205, -0.8703) -> (-4.3182, -0.8572)
  line L1526 (-4.3182, -0.8572) -> (-4.3194, -0.8383)
  line L1527 (-4.3194, -0.8383) -> (-4.3458, -0.6883)
  line L1528 (-4.3458, -0.6883) -> (-4.3671, -0.5375)
  line L1529 (-4.3671, -0.5375) -> (-4.3718, -0.5191)
  line L1530 (-4.3718, -0.5191) -> (-4.378, -0.5074)
  line L1531 (-4.378, -0.5074) -> (-4.3865, -0.4962)
  line L1532 (-4.3865, -0.4962) -> (-4.3975, -0.4856)
  line L1533 (-4.3975, -0.4856) -> (-4.4108, -0.4758)
  line L1534 (-4.4108, -0.4758) -> (-4.4264, -0.4668)
  line L1535 (-4.4264, -0.4668) -> (-4.4444, -0.4587)
  line L1536 (-4.4444, -0.4587) -> (-4.4646, -0.4516)
  line L1537 (-4.4646, -0.4516) -> (-4.487, -0.4455)
  line L1538 (-4.487, -0.4455) -> (-4.5117, -0.4407)
  line L1539 (-4.5117, -0.4407) -> (-4.5385, -0.4371)
  line L1540 (-4.5385, -0.4371) -> (-4.5984, -0.4341)
  line L1541 (-4.5984, -0.4341) -> (-4.6862, -0.4388)
  line L1542 (-4.6862, -0.4388) -> (-4.7327, -0.438)
  line L1543 (-4.7327, -0.438) -> (-4.8085, -0.43)
  line L1544 (-4.8085, -0.43) -> (-4.8574, -0.422)
  line L1545 (-4.8574, -0.422) -> (-4.9147, -0.41)
  line L1546 (-4.9147, -0.41) -> (-4.9802, -0.3935)
  line L1547 (-4.9802, -0.3935) -> (-5.0516, -0.3723)
  line L1548 (-5.0516, -0.3723) -> (-5.1313, -0.3449)
  line L1549 (-5.1313, -0.3449) -> (-5.2159, -0.3118)
  line L1550 (-5.2159, -0.3118) -> (-5.3081, -0.2712)
  line L1551 (-5.3081, -0.2712) -> (-5.4053, -0.2235)
  line L1552 (-5.4053, -0.2235) -> (-5.4973, -0.1736)
  arc A32 (-5.4973, 0.1736) -> (-5.4973, -0.1736) centre (0, 0) ccw
  line L1553 (-5.4973, 0.1736) -> (-5.4053, 0.2235)
  line L1554 (-5.4053, 0.2235) -> (-5.3081, 0.2712)
  line L1555 (-5.3081, 0.2712) -> (-5.2159, 0.3118)
  line L1556 (-5.2159, 0.3118) -> (-5.1313, 0.3449)
  line L1557 (-5.1313, 0.3449) -> (-5.0516, 0.3723)
  line L1558 (-5.0516, 0.3723) -> (-4.9802, 0.3935)
  line L1559 (-4.9802, 0.3935) -> (-4.9147, 0.41)
  line L1560 (-4.9147, 0.41) -> (-4.8574, 0.422)
  line L1561 (-4.8574, 0.422) -> (-4.8085, 0.43)
  line L1562 (-4.8085, 0.43) -> (-4.7327, 0.438)
  line L1563 (-4.7327, 0.438) -> (-4.6862, 0.4388)
  line L1564 (-4.6862, 0.4388) -> (-4.5984, 0.4341)
  line L1565 (-4.5984, 0.4341) -> (-4.5385, 0.4371)
  line L1566 (-4.5385, 0.4371) -> (-4.5117, 0.4407)
  line L1567 (-4.5117, 0.4407) -> (-4.487, 0.4455)
  line L1568 (-4.487, 0.4455) -> (-4.4646, 0.4516)
  line L1569 (-4.4646, 0.4516) -> (-4.4444, 0.4587)
  line L1570 (-4.4444, 0.4587) -> (-4.4264, 0.4668)
  line L1571 (-4.4264, 0.4668) -> (-4.4108, 0.4758)
  line L1572 (-4.4108, 0.4758) -> (-4.3975, 0.4856)
  line L1573 (-4.3975, 0.4856) -> (-4.3865, 0.4962)
  line L1574 (-4.3865, 0.4962) -> (-4.378, 0.5074)
  line L1575 (-4.378, 0.5074) -> (-4.3718, 0.5191)
  line L1576 (-4.3718, 0.5191) -> (-4.3671, 0.5375)
  line L1577 (-4.3671, 0.5375) -> (-4.3458, 0.6883)
  line L1578 (-4.3458, 0.6883) -> (-4.3194, 0.8383)
  line L1579 (-4.3194, 0.8383) -> (-4.3182, 0.8572)
  line L1580 (-4.3182, 0.8572) -> (-4.3205, 0.8703)
  line L1581 (-4.3205, 0.8703) -> (-4.3252, 0.8836)
  line L1582 (-4.3252, 0.8836) -> (-4.3323, 0.897)
  line L1583 (-4.3323, 0.897) -> (-4.3419, 0.9105)
  line L1584 (-4.3419, 0.9105) -> (-4.354, 0.9239)
  line L1585 (-4.354, 0.9239) -> (-4.3686, 0.9372)
  line L1586 (-4.3686, 0.9372) -> (-4.3856, 0.9502)
  line L1587 (-4.3856, 0.9502) -> (-4.4051, 0.9628)
  line L1588 (-4.4051, 0.9628) -> (-4.427, 0.9751)
  line L1589 (-4.427, 0.9751) -> (-4.4514, 0.9867)
  line L1590 (-4.4514, 0.9867) -> (-4.5075, 1.0081)
  line L1591 (-4.5075, 1.0081) -> (-4.5924, 1.0307)
  line L1592 (-4.5924, 1.0307) -> (-4.6364, 1.046)
  line L1593 (-4.6364, 1.046) -> (-4.7061, 1.0769)
  line L1594 (-4.7061, 1.0769) -> (-4.75, 1.0997)
  line L1595 (-4.75, 1.0997) -> (-4.8009, 1.1288)
  line L1596 (-4.8009, 1.1288) -> (-4.8581, 1.1647)
  line L1597 (-4.8581, 1.1647) -> (-4.9194, 1.207)
  line L1598 (-4.9194, 1.207) -> (-4.9868, 1.2577)
  line L1599 (-4.9868, 1.2577) -> (-5.0569, 1.3152)
  line L1600 (-5.0569, 1.3152) -> (-5.1322, 1.3823)
  line L1601 (-5.1322, 1.3823) -> (-5.2098, 1.4578)
  line L1602 (-5.2098, 1.4578) -> (-5.2818, 1.5336)
  arc A33 (-5.1745, 1.8639) -> (-5.2818, 1.5336) centre (0, 0) ccw
  line L1603 (-5.1745, 1.8639) -> (-5.0717, 1.8829)
  line L1604 (-5.0717, 1.8829) -> (-4.9645, 1.8983)
  line L1605 (-4.9645, 1.8983) -> (-4.8642, 1.9084)
  line L1606 (-4.8642, 1.9084) -> (-4.7736, 1.9137)
  line L1607 (-4.7736, 1.9137) -> (-4.6893, 1.9151)
  line L1608 (-4.6893, 1.9151) -> (-4.6149, 1.9132)
  line L1609 (-4.6149, 1.9132) -> (-4.5475, 1.9087)
  line L1610 (-4.5475, 1.9087) -> (-4.4892, 1.9023)
  line L1611 (-4.4892, 1.9023) -> (-4.4403, 1.8949)
  line L1612 (-4.4403, 1.8949) -> (-4.3657, 1.879)
  line L1613 (-4.3657, 1.879) -> (-4.3212, 1.8655)
  line L1614 (-4.3212, 1.8655) -> (-4.2391, 1.8339)
  line L1615 (-4.2391, 1.8339) -> (-4.1813, 1.8182)
  line L1616 (-4.1813, 1.8182) -> (-4.1547, 1.8133)
  line L1617 (-4.1547, 1.8133) -> (-4.1297, 1.8103)
  line L1618 (-4.1297, 1.8103) -> (-4.1065, 1.8091)
  line L1619 (-4.1065, 1.8091) -> (-4.0851, 1.8096)
  line L1620 (-4.0851, 1.8096) -> (-4.0655, 1.8118)
  line L1621 (-4.0655, 1.8118) -> (-4.0479, 1.8155)
  line L1622 (-4.0479, 1.8155) -> (-4.0322, 1.8208)
  line L1623 (-4.0322, 1.8208) -> (-4.0185, 1.8274)
  line L1624 (-4.0185, 1.8274) -> (-4.0069, 1.8354)
  line L1625 (-4.0069, 1.8354) -> (-3.9974, 1.8447)
  line L1626 (-3.9974, 1.8447) -> (-3.9872, 1.8607)
  line L1627 (-3.9872, 1.8607) -> (-3.9204, 1.9976)
  line L1628 (-3.9204, 1.9976) -> (-3.8489, 2.1321)
  line L1629 (-3.8489, 2.1321) -> (-3.842, 2.1497)
  line L1630 (-3.842, 2.1497) -> (-3.8401, 2.1628)
  line L1631 (-3.8401, 2.1628) -> (-3.8404, 2.1769)
  line L1632 (-3.8404, 2.1769) -> (-3.8431, 2.1919)
  line L1633 (-3.8431, 2.1919) -> (-3.8481, 2.2077)
  line L1634 (-3.8481, 2.2077) -> (-3.8554, 2.2242)
  line L1635 (-3.8554, 2.2242) -> (-3.8652, 2.2413)
  line L1636 (-3.8652, 2.2413) -> (-3.8773, 2.2589)
  line L1637 (-3.8773, 2.2589) -> (-3.892, 2.277)
  line L1638 (-3.892, 2.277) -> (-3.9091, 2.2954)
  line L1639 (-3.9091, 2.2954) -> (-3.9286, 2.314)
  line L1640 (-3.9286, 2.314) -> (-3.9753, 2.3516)
  line L1641 (-3.9753, 2.3516) -> (-4.0491, 2.3994)
  line L1642 (-4.0491, 2.3994) -> (-4.0862, 2.4275)
  line L1643 (-4.0862, 2.4275) -> (-4.1429, 2.4785)
  line L1644 (-4.1429, 2.4785) -> (-4.1777, 2.5137)
  line L1645 (-4.1777, 2.5137) -> (-4.2171, 2.5571)
  line L1646 (-4.2171, 2.5571) -> (-4.2604, 2.609)
  line L1647 (-4.2604, 2.609) -> (-4.3057, 2.6681)
  line L1648 (-4.3057, 2.6681) -> (-4.3541, 2.7371)
  line L1649 (-4.3541, 2.7371) -> (-4.403, 2.8135)
  line L1650 (-4.403, 2.8135) -> (-4.4538, 2.9006)
  line L1651 (-4.4538, 2.9006) -> (-4.5044, 2.9964)
  line L1652 (-4.5044, 2.9964) -> (-4.5494, 3.0907)
  arc A34 (-4.3453, 3.3717) -> (-4.5494, 3.0907) centre (0, 0) ccw
  line L1653 (-4.3453, 3.3717) -> (-4.2416, 3.358)
  line L1654 (-4.2416, 3.358) -> (-4.1349, 3.3395)
  line L1655 (-4.1349, 3.3395) -> (-4.0364, 3.3181)
  line L1656 (-4.0364, 3.3181) -> (-3.9486, 3.2952)
  line L1657 (-3.9486, 3.2952) -> (-3.868, 3.2704)
  line L1658 (-3.868, 3.2704) -> (-3.7978, 3.2457)
  line L1659 (-3.7978, 3.2457) -> (-3.7351, 3.2205)
  line L1660 (-3.7351, 3.2205) -> (-3.6817, 3.1965)
  line L1661 (-3.6817, 3.1965) -> (-3.6374, 3.1743)
  line L1662 (-3.6374, 3.1743) -> (-3.5714, 3.1361)
  line L1663 (-3.5714, 3.1361) -> (-3.5332, 3.1095)
  line L1664 (-3.5332, 3.1095) -> (-3.465, 3.0541)
  line L1665 (-3.465, 3.0541) -> (-3.4148, 3.0213)
  line L1666 (-3.4148, 3.0213) -> (-3.391, 3.0084)
  line L1667 (-3.391, 3.0084) -> (-3.3682, 2.9979)
  line L1668 (-3.3682, 2.9979) -> (-3.3465, 2.9895)
  line L1669 (-3.3465, 2.9895) -> (-3.326, 2.9834)
  line L1670 (-3.326, 2.9834) -> (-3.3067, 2.9794)
  line L1671 (-3.3067, 2.9794) -> (-3.2887, 2.9775)
  line L1672 (-3.2887, 2.9775) -> (-3.2722, 2.9777)
  line L1673 (-3.2722, 2.9777) -> (-3.2571, 2.9798)
  line L1674 (-3.2571, 2.9798) -> (-3.2436, 2.9838)
  line L1675 (-3.2436, 2.9838) -> (-3.2317, 2.9896)
  line L1676 (-3.2317, 2.9896) -> (-3.2171, 3.0017)
  line L1677 (-3.2171, 3.0017) -> (-3.1113, 3.1113)
  line L1678 (-3.1113, 3.1113) -> (-3.0017, 3.2171)
  line L1679 (-3.0017, 3.2171) -> (-2.9896, 3.2317)
  line L1680 (-2.9896, 3.2317) -> (-2.9838, 3.2436)
  line L1681 (-2.9838, 3.2436) -> (-2.9798, 3.2571)
  line L1682 (-2.9798, 3.2571) -> (-2.9777, 3.2722)
  line L1683 (-2.9777, 3.2722) -> (-2.9775, 3.2887)
  line L1684 (-2.9775, 3.2887) -> (-2.9794, 3.3067)
  line L1685 (-2.9794, 3.3067) -> (-2.9834, 3.326)
  line L1686 (-2.9834, 3.326) -> (-2.9895, 3.3465)
  line L1687 (-2.9895, 3.3465) -> (-2.9979, 3.3682)
  line L1688 (-2.9979, 3.3682) -> (-3.0084, 3.391)
  line L1689 (-3.0084, 3.391) -> (-3.0213, 3.4148)
  line L1690 (-3.0213, 3.4148) -> (-3.0541, 3.465)
  line L1691 (-3.0541, 3.465) -> (-3.1095, 3.5332)
  line L1692 (-3.1095, 3.5332) -> (-3.1361, 3.5714)
  line L1693 (-3.1361, 3.5714) -> (-3.1743, 3.6374)
  line L1694 (-3.1743, 3.6374) -> (-3.1965, 3.6817)
  line L1695 (-3.1965, 3.6817) -> (-3.2205, 3.7351)
  line L1696 (-3.2205, 3.7351) -> (-3.2457, 3.7978)
  line L1697 (-3.2457, 3.7978) -> (-3.2704, 3.868)
  line L1698 (-3.2704, 3.868) -> (-3.2952, 3.9486)
  line L1699 (-3.2952, 3.9486) -> (-3.3181, 4.0364)
  line L1700 (-3.3181, 4.0364) -> (-3.3395, 4.1349)
  line L1701 (-3.3395, 4.1349) -> (-3.358, 4.2416)
  line L1702 (-3.358, 4.2416) -> (-3.3717, 4.3453)
  arc A35 (-3.0907, 4.5494) -> (-3.3717, 4.3453) centre (0, 0) ccw
  line L1703 (-3.0907, 4.5494) -> (-2.9964, 4.5044)
  line L1704 (-2.9964, 4.5044) -> (-2.9006, 4.4538)
  line L1705 (-2.9006, 4.4538) -> (-2.8135, 4.403)
  line L1706 (-2.8135, 4.403) -> (-2.7371, 4.3541)
  line L1707 (-2.7371, 4.3541) -> (-2.6681, 4.3057)
  line L1708 (-2.6681, 4.3057) -> (-2.609, 4.2604)
  line L1709 (-2.609, 4.2604) -> (-2.5571, 4.2171)
  line L1710 (-2.5571, 4.2171) -> (-2.5137, 4.1777)
  line L1711 (-2.5137, 4.1777) -> (-2.4785, 4.1429)
  line L1712 (-2.4785, 4.1429) -> (-2.4275, 4.0862)
  line L1713 (-2.4275, 4.0862) -> (-2.3994, 4.0491)
  line L1714 (-2.3994, 4.0491) -> (-2.3516, 3.9753)
  line L1715 (-2.3516, 3.9753) -> (-2.314, 3.9286)
  line L1716 (-2.314, 3.9286) -> (-2.2954, 3.9091)
  line L1717 (-2.2954, 3.9091) -> (-2.277, 3.892)
  line L1718 (-2.277, 3.892) -> (-2.2589, 3.8773)
  line L1719 (-2.2589, 3.8773) -> (-2.2413, 3.8652)
  line L1720 (-2.2413, 3.8652) -> (-2.2242, 3.8554)
  line L1721 (-2.2242, 3.8554) -> (-2.2077, 3.8481)
  line L1722 (-2.2077, 3.8481) -> (-2.1919, 3.8431)
  line L1723 (-2.1919, 3.8431) -> (-2.1769, 3.8404)
  line L1724 (-2.1769, 3.8404) -> (-2.1628, 3.8401)
  line L1725 (-2.1628, 3.8401) -> (-2.1497, 3.842)
  line L1726 (-2.1497, 3.842) -> (-2.1321, 3.8489)
  line L1727 (-2.1321, 3.8489) -> (-1.9976, 3.9204)
  line L1728 (-1.9976, 3.9204) -> (-1.8607, 3.9872)
  line L1729 (-1.8607, 3.9872) -> (-1.8447, 3.9974)
  line L1730 (-1.8447, 3.9974) -> (-1.8354, 4.0069)
  line L1731 (-1.8354, 4.0069) -> (-1.8274, 4.0185)
  line L1732 (-1.8274, 4.0185) -> (-1.8208, 4.0322)
  line L1733 (-1.8208, 4.0322) -> (-1.8155, 4.0479)
  line L1734 (-1.8155, 4.0479) -> (-1.8118, 4.0655)
  line L1735 (-1.8118, 4.0655) -> (-1.8096, 4.0851)
  line L1736 (-1.8096, 4.0851) -> (-1.8091, 4.1065)
  line L1737 (-1.8091, 4.1065) -> (-1.8103, 4.1297)
  line L1738 (-1.8103, 4.1297) -> (-1.8133, 4.1547)
  line L1739 (-1.8133, 4.1547) -> (-1.8182, 4.1813)
  line L1740 (-1.8182, 4.1813) -> (-1.8339, 4.2391)
  line L1741 (-1.8339, 4.2391) -> (-1.8655, 4.3212)
  line L1742 (-1.8655, 4.3212) -> (-1.879, 4.3657)
  line L1743 (-1.879, 4.3657) -> (-1.8949, 4.4403)
  line L1744 (-1.8949, 4.4403) -> (-1.9023, 4.4892)
  line L1745 (-1.9023, 4.4892) -> (-1.9087, 4.5475)
  line L1746 (-1.9087, 4.5475) -> (-1.9132, 4.6149)
  line L1747 (-1.9132, 4.6149) -> (-1.9151, 4.6893)
  line L1748 (-1.9151, 4.6893) -> (-1.9137, 4.7736)
  line L1749 (-1.9137, 4.7736) -> (-1.9084, 4.8642)
  line L1750 (-1.9084, 4.8642) -> (-1.8983, 4.9645)
  line L1751 (-1.8983, 4.9645) -> (-1.8829, 5.0717)
  line L1752 (-1.8829, 5.0717) -> (-1.8639, 5.1745)
  arc A36 (-1.5336, 5.2818) -> (-1.8639, 5.1745) centre (0, 0) ccw
  line L1753 (-1.5336, 5.2818) -> (-1.4578, 5.2098)
  line L1754 (-5.2818, -1.5336) -> (-5.2098, -1.4578)
  line L1755 (-1.3823, 5.1322) -> (-1.3152, 5.0569)
  line L1756 (-1.3152, 5.0569) -> (-1.2577, 4.9868)
  line L1757 (-1.2577, 4.9868) -> (-1.207, 4.9194)
  line L1758 (-1.207, 4.9194) -> (-1.1647, 4.8581)
  line L1759 (-1.1647, 4.8581) -> (-1.1288, 4.8009)
  line L1760 (-1.1288, 4.8009) -> (-1.0997, 4.75)
  line L1761 (-1.0997, 4.75) -> (-1.0769, 4.7061)
  line L1762 (-1.0769, 4.7061) -> (-1.046, 4.6364)
  line L1763 (-1.046, 4.6364) -> (-1.0307, 4.5924)
  line L1764 (-1.0307, 4.5924) -> (-1.0081, 4.5075)
  line L1765 (-1.0081, 4.5075) -> (-0.9867, 4.4514)
  line L1766 (-0.9867, 4.4514) -> (-0.9751, 4.427)
  line L1767 (-0.9751, 4.427) -> (-0.9628, 4.4051)
  line L1768 (-0.9628, 4.4051) -> (-0.9502, 4.3856)
  line L1769 (-0.9502, 4.3856) -> (-0.9372, 4.3686)
  line L1770 (-0.9372, 4.3686) -> (-0.9239, 4.354)
  line L1771 (-0.9239, 4.354) -> (-0.9105, 4.3419)
  line L1772 (-0.9105, 4.3419) -> (-0.897, 4.3323)
  line L1773 (-0.897, 4.3323) -> (-0.8836, 4.3252)
  line L1774 (-0.8836, 4.3252) -> (-0.8703, 4.3205)
  line L1775 (-0.8703, 4.3205) -> (-0.8572, 4.3182)
  line L1776 (-0.8572, 4.3182) -> (-0.8383, 4.3194)
  line L1777 (-0.8383, 4.3194) -> (-0.6883, 4.3458)
  line L1778 (-0.6883, 4.3458) -> (-0.5375, 4.3671)
  line L1779 (-0.5375, 4.3671) -> (-0.5191, 4.3718)
  line L1780 (-0.5191, 4.3718) -> (-0.5074, 4.378)
  line L1781 (-0.5074, 4.378) -> (-0.4962, 4.3865)
  line L1782 (-0.4962, 4.3865) -> (-0.4856, 4.3975)
  line L1783 (-0.4856, 4.3975) -> (-0.4758, 4.4108)
  line L1784 (-0.4758, 4.4108) -> (-0.4668, 4.4264)
  line L1785 (-0.4668, 4.4264) -> (-0.4587, 4.4444)
  line L1786 (-0.4587, 4.4444) -> (-0.4516, 4.4646)
  line L1787 (-0.4516, 4.4646) -> (-0.4455, 4.487)
  line L1788 (-0.4455, 4.487) -> (-0.4407, 4.5117)
  line L1789 (-0.4407, 4.5117) -> (-0.4371, 4.5385)
  line L1790 (-0.4371, 4.5385) -> (-0.4341, 4.5984)
  line L1791 (-0.4341, 4.5984) -> (-0.4388, 4.6862)
  line L1792 (-0.4388, 4.6862) -> (-0.438, 4.7327)
  line L1793 (-0.438, 4.7327) -> (-0.43, 4.8085)
  line L1794 (-0.43, 4.8085) -> (-0.422, 4.8574)
  line L1795 (-0.422, 4.8574) -> (-0.41, 4.9147)
  line L1796 (-0.41, 4.9147) -> (-0.3935, 4.9802)
  line L1797 (-0.3935, 4.9802) -> (-0.3723, 5.0516)
  line L1798 (-0.3723, 5.0516) -> (-0.3449, 5.1313)
  line L1799 (-0.3449, 5.1313) -> (-0.3118, 5.2159)
  line L1800 (-0.3118, 5.2159) -> (-0.2712, 5.3081)
  line L1801 (-0.2712, 5.3081) -> (-0.2235, 5.4053)
  line L1802 (-0.2235, 5.4053) -> (-0.1736, 5.4973)
  arc A37 (0.1736, 5.4973) -> (-0.1736, 5.4973) centre (0, 0) ccw
  line L1803 (0.1736, 5.4973) -> (0.2235, 5.4053)
  line L1804 (0.2235, 5.4053) -> (0.2712, 5.3081)
  line L1805 (0.2712, 5.3081) -> (0.3118, 5.2159)
  line L1806 (0.3118, 5.2159) -> (0.3449, 5.1313)
  line L1807 (0.3449, 5.1313) -> (0.3723, 5.0516)
  line L1808 (0.3723, 5.0516) -> (0.3935, 4.9802)
  line L1809 (0.3935, 4.9802) -> (0.41, 4.9147)
  line L1810 (0.41, 4.9147) -> (0.422, 4.8574)
  line L1811 (0.422, 4.8574) -> (0.43, 4.8085)
  line L1812 (0.43, 4.8085) -> (0.438, 4.7327)
  line L1813 (0.438, 4.7327) -> (0.4388, 4.6862)
  line L1814 (0.4388, 4.6862) -> (0.4341, 4.5984)
  line L1815 (0.4341, 4.5984) -> (0.4371, 4.5385)
  line L1816 (0.4371, 4.5385) -> (0.4407, 4.5117)
  line L1817 (0.4407, 4.5117) -> (0.4455, 4.487)
  line L1818 (0.4455, 4.487) -> (0.4516, 4.4646)
  line L1819 (0.4516, 4.4646) -> (0.4587, 4.4444)
  line L1820 (0.4587, 4.4444) -> (0.4668, 4.4264)
  line L1821 (0.4668, 4.4264) -> (0.4758, 4.4108)
  line L1822 (0.4758, 4.4108) -> (0.4856, 4.3975)
  line L1823 (0.4856, 4.3975) -> (0.4962, 4.3865)
  line L1824 (0.4962, 4.3865) -> (0.5074, 4.378)
  line L1825 (0.5074, 4.378) -> (0.5191, 4.3718)
  line L1826 (0.5191, 4.3718) -> (0.5375, 4.3671)
  line L1827 (0.5375, 4.3671) -> (0.6883, 4.3458)
  line L1828 (0.6883, 4.3458) -> (0.8383, 4.3194)
  line L1829 (0.8383, 4.3194) -> (0.8572, 4.3182)
  line L1830 (0.8572, 4.3182) -> (0.8703, 4.3205)
  line L1831 (0.8703, 4.3205) -> (0.8836, 4.3252)
  line L1832 (0.8836, 4.3252) -> (0.897, 4.3323)
  line L1833 (0.897, 4.3323) -> (0.9105, 4.3419)
  line L1834 (0.9105, 4.3419) -> (0.9239, 4.354)
  line L1835 (0.9239, 4.354) -> (0.9372, 4.3686)
  line L1836 (0.9372, 4.3686) -> (0.9502, 4.3856)
  line L1837 (0.9502, 4.3856) -> (0.9628, 4.4051)
  line L1838 (0.9628, 4.4051) -> (0.9751, 4.427)
  line L1839 (0.9751, 4.427) -> (0.9867, 4.4514)
  line L1840 (0.9867, 4.4514) -> (1.0081, 4.5075)
  line L1841 (1.0081, 4.5075) -> (1.0307, 4.5924)
  line L1842 (1.0307, 4.5924) -> (1.046, 4.6364)
  line L1843 (1.046, 4.6364) -> (1.0769, 4.7061)
  line L1844 (1.0769, 4.7061) -> (1.0997, 4.75)
  line L1845 (1.0997, 4.75) -> (1.1288, 4.8009)
  line L1846 (1.1288, 4.8009) -> (1.1647, 4.8581)
  line L1847 (1.1647, 4.8581) -> (1.207, 4.9194)
  line L1848 (1.207, 4.9194) -> (1.2577, 4.9868)
  line L1849 (1.2577, 4.9868) -> (1.3152, 5.0569)
  line L1850 (1.3152, 5.0569) -> (1.3823, 5.1322)
  line L1851 (1.3823, 5.1322) -> (1.4578, 5.2098)
  line L1852 (1.4578, 5.2098) -> (1.5336, 5.2818)
  arc A38 (1.8639, 5.1745) -> (1.5336, 5.2818) centre (0, 0) ccw
  line L1853 (1.8639, 5.1745) -> (1.8829, 5.0717)
  line L1854 (1.8829, 5.0717) -> (1.8983, 4.9645)
  line L1855 (1.8983, 4.9645) -> (1.9084, 4.8642)
  line L1856 (1.9084, 4.8642) -> (1.9137, 4.7736)
  line L1857 (1.9137, 4.7736) -> (1.9151, 4.6893)
  line L1858 (1.9151, 4.6893) -> (1.9132, 4.6149)
  line L1859 (1.9132, 4.6149) -> (1.9087, 4.5475)
  line L1860 (1.9087, 4.5475) -> (1.9023, 4.4892)
  line L1861 (1.9023, 4.4892) -> (1.8949, 4.4403)
  line L1862 (1.8949, 4.4403) -> (1.879, 4.3657)
  line L1863 (1.879, 4.3657) -> (1.8655, 4.3212)
  line L1864 (1.8655, 4.3212) -> (1.8339, 4.2391)
  line L1865 (1.8339, 4.2391) -> (1.8182, 4.1813)
  line L1866 (1.8182, 4.1813) -> (1.8133, 4.1547)
  line L1867 (1.8133, 4.1547) -> (1.8103, 4.1297)
  line L1868 (1.8103, 4.1297) -> (1.8091, 4.1065)
  line L1869 (1.8091, 4.1065) -> (1.8096, 4.0851)
  line L1870 (1.8096, 4.0851) -> (1.8118, 4.0655)
  line L1871 (1.8118, 4.0655) -> (1.8155, 4.0479)
  line L1872 (1.8155, 4.0479) -> (1.8208, 4.0322)
  line L1873 (1.8208, 4.0322) -> (1.8274, 4.0185)
  line L1874 (1.8274, 4.0185) -> (1.8354, 4.0069)
  line L1875 (1.8354, 4.0069) -> (1.8447, 3.9974)
  line L1876 (1.8447, 3.9974) -> (1.8607, 3.9872)
  line L1877 (1.8607, 3.9872) -> (1.9976, 3.9204)
  line L1878 (1.9976, 3.9204) -> (2.1321, 3.8489)
  line L1879 (2.1321, 3.8489) -> (2.1497, 3.842)
  line L1880 (2.1497, 3.842) -> (2.1628, 3.8401)
  line L1881 (2.1628, 3.8401) -> (2.1769, 3.8404)
  line L1882 (2.1769, 3.8404) -> (2.1919, 3.8431)
  line L1883 (2.1919, 3.8431) -> (2.2077, 3.8481)
  line L1884 (2.2077, 3.8481) -> (2.2242, 3.8554)
  line L1885 (2.2242, 3.8554) -> (2.2413, 3.8652)
  line L1886 (2.2413, 3.8652) -> (2.2589, 3.8773)
  line L1887 (2.2589, 3.8773) -> (2.277, 3.892)
  line L1888 (2.277, 3.892) -> (2.2954, 3.9091)
  line L1889 (2.2954, 3.9091) -> (2.314, 3.9286)
  line L1890 (2.314, 3.9286) -> (2.3516, 3.9753)
  line L1891 (2.3516, 3.9753) -> (2.3994, 4.0491)
  line L1892 (2.3994, 4.0491) -> (2.4275, 4.0862)
  line L1893 (2.4275, 4.0862) -> (2.4785, 4.1429)